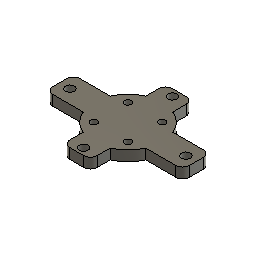
Base_Part1 (Autodesk Fusion 360 design; units mm, degrees)
part number: 2025-04-16-17-35-49-953
Autodesk Fusion 360 part; units mm, degrees
note: some values were not read from the file. Set by a fixed rule: which sketch regions a step uses.
sketch "Sketch1" plane through (0, 0, 0) normal (0, 1, 0) x (1, 0, 0)
  line L0 (20, 75) -> (-20, 75)
  line L1 (-100, 20) -> (-100, -20)
  line L2 (-20, -75) -> (20, -75)
  line L3 (100, -20) -> (100, 20)
  line L4 (20, 45.8258) -> (20, 75)
  line L5 (20, 75) -> (-20, 75)
  line L6 (-20, 75) -> (-20, 45.8258)
  line L7 (20, -45.8258) -> (20, -75)
  line L8 (20, -75) -> (-20, -75)
  line L9 (-20, -75) -> (-20, -45.8258)
  line L10 (45.8258, 20) -> (100, 20)
  line L11 (100, 20) -> (100, -20)
  line L12 (100, -20) -> (45.8258, -20)
  line L13 (-45.8258, 20) -> (-100, 20)
  line L14 (-100, 20) -> (-100, -20)
  arc A0 (45.8258, 20) -> (20, 45.8258) centre (0, 0) ccw
  arc A1 (-20, 45.8258) -> (-45.8258, 20) centre (0, 0) ccw
  line L15 (-100, -20) -> (-45.8258, -20)
  arc A2 (-45.8258, -20) -> (-20, -45.8258) centre (0, 0) ccw
  arc A3 (20, -45.8258) -> (45.8258, -20) centre (0, 0) ccw
  dimension "d70" = 100
  constraint horizontal L0
  constraint perpendicular L0 L1
  constraint parallel L0 L2
  constraint parallel L1 L3
  constraint coincident A0.centre A1.centre
  constraint vertical L4
  constraint horizontal L5
  constraint vertical L6
  constraint vertical L7
  constraint horizontal L8
  constraint vertical L9
  constraint horizontal L10
  constraint vertical L11
  constraint horizontal L12
  constraint horizontal L13
  constraint vertical L14
  constraint horizontal L15
  constraint coincident L10.start A1
  constraint concentric A0 A1
  constraint concentric A1 A2
  constraint concentric A2 A3
  measures "d70" diameter of A1
extrude "Extrude1" add sketch "Sketch1" along normal blind 15
sketch "Sketch3" plane through (0, 15, 0) normal (0, 1, 0) x (-1, 0, 0)
  line L0 (-20, 75) -> (-20, 45.8258)
  line L1 (-45.8258, 20) -> (-100, 20)
  line L2 (-100, 20) -> (-100, -20)
  line L3 (-100, -20) -> (-45.8258, -20)
  line L4 (-20, -45.8258) -> (-20, -75)
  line L5 (-20, -75) -> (20, -75)
  line L6 (20, -75) -> (20, -45.8258)
  line L7 (45.8258, -20) -> (100, -20)
  line L8 (100, -20) -> (100, 20)
  line L9 (100, 20) -> (45.8258, 20)
  line L10 (20, 45.8258) -> (20, 75)
  line L11 (20, 75) -> (-20, 75)
  circle A0 centre (0, 0) radius 50
  arc A1 (-20, 45.8258) -> (-45.8258, 20) centre (0, 0) ccw
  arc A2 (-45.8258, -20) -> (-20, -45.8258) centre (0, 0) ccw
  arc A3 (20, -45.8258) -> (45.8258, -20) centre (0, 0) ccw
  arc A4 (45.8258, 20) -> (20, 45.8258) centre (0, 0) ccw
  dimension "d71" = 100
  constraint coincident A0.centre A1.centre
  measures "d71" diameter of A0
sketch "Sketch4" plane through (0, 15, 0) normal (0, 1, 0) x (-1, 0, 0)
  line L0 (45.8258, -20) -> (100, -20)
  line L1 (100, -20) -> (100, 20)
  line L2 (100, 20) -> (45.8258, 20)
  circle A0 centre (0, -65) radius 6.5
  circle A1 centre (0, 65) radius 6.5
  circle A2 centre (-85, 0) radius 6.5
  circle A3 centre (85, 0) radius 6.5
  line L3 (-20, 75) -> (-20, 45.8258)
  arc A4 (-20, 45.8258) -> (-45.8258, 20) centre (0, 0) ccw
  line L4 (-45.8258, 20) -> (-100, 20)
  line L5 (-100, 20) -> (-100, -20)
  line L6 (-100, -20) -> (-45.8258, -20)
  arc A5 (-45.8258, -20) -> (-20, -45.8258) centre (0, 0) ccw
  line L7 (-20, -45.8258) -> (-20, -75)
  line L8 (-20, -75) -> (20, -75)
  line L9 (20, -75) -> (20, -45.8258)
  arc A6 (20, -45.8258) -> (45.8258, -20) centre (0, 0) ccw
  arc A7 (45.8258, 20) -> (20, 45.8258) centre (0, 0) ccw
  line L10 (20, 45.8258) -> (20, 75)
  line L11 (20, 75) -> (-20, 75)
  dimension "d30" = 13
  dimension "d31" = 13
  dimension "d32" = 13
  dimension "d33" = 13
  measures "d30" diameter of A0
  measures "d31" diameter of A1
  measures "d32" diameter of A2
  measures "d33" diameter of A3
extrude "Extrude3" cut sketch "Sketch4" against normal blind 15 contours A0 | A1 | A2 | A3
fillet "Fillet11" radius 10 1 edges at (20, 7.5, 75)
fillet "Fillet12" radius 10 7 edges at (100, 7.5, 20) (100, 7.5, -20) (20, 7.5, -75) (-100, 7.5, 20) (-20, 7.5, 75) (-20, 7.5, -75) (-100, 7.5, -20)
sketch "Sketch11" plane through (0, 15, 0) normal (0, 1, 0) x (-1, 0, 0)
  circle A0 centre (0, -65) radius 6.5
  circle A1 centre (-85, 0) radius 6.5
  circle A2 centre (85, 0) radius 6.5
  circle A3 centre (0, 65) radius 6.5
  arc A4 (90, -20) -> (100, -10) centre (90, -10) ccw
  line L0 (100, -10) -> (100, 10)
  arc A5 (100, 10) -> (90, 20) centre (90, 10) ccw
  line L1 (90, 20) -> (45.8258, 20)
  arc A6 (45.8258, 20) -> (20, 45.8258) centre (0, 0) ccw
  line L2 (20, 45.8258) -> (20, 65)
  arc A7 (20, 65) -> (10, 75) centre (10, 65) ccw
  line L3 (10, 75) -> (-10, 75)
  arc A8 (-10, 75) -> (-20, 65) centre (-10, 65) ccw
  line L4 (-20, 65) -> (-20, 45.8258)
  arc A9 (-20, 45.8258) -> (-45.8258, 20) centre (0, 0) ccw
  line L5 (-45.8258, 20) -> (-90, 20)
  arc A10 (-90, 20) -> (-100, 10) centre (-90, 10) ccw
  line L6 (-100, 10) -> (-100, -10)
  arc A11 (-100, -10) -> (-90, -20) centre (-90, -10) ccw
  line L7 (-90, -20) -> (-45.8258, -20)
  arc A12 (-45.8258, -20) -> (-20, -45.8258) centre (0, 0) ccw
  line L8 (-20, -45.8258) -> (-20, -65)
  arc A13 (-20, -65) -> (-10, -75) centre (-10, -65) ccw
  line L9 (-10, -75) -> (10, -75)
  arc A14 (10, -75) -> (20, -65) centre (10, -65) ccw
  line L10 (20, -65) -> (20, -45.8258)
  arc A15 (20, -45.8258) -> (45.8258, -20) centre (0, 0) ccw
  line L11 (45.8258, -20) -> (90, -20)
  line L12 (0, 0) -> (50, -50)
  line L13 (0, 0) -> (63.8718, 0) construction
  circle A16 centre (25, -25) radius 5
  circle A17 centre (25, 25) radius 5
  circle A18 centre (-25, 25) radius 5
  circle A19 centre (-25, -25) radius 5
  dimension "d77" = 45
  dimension "d78" = 10
  dimension "d79" = 25
  dimension "d81" = 360
  constraint horizontal L13
  constraint coincident A6.centre A9.centre
  constraint midpoint L12 A16.centre
  measures "d77" angle of L12 L13
  measures "d78" diameter of A16
  measures "d79" horizontal distance of A6.centre A16.centre
extrude "Extrude10" cut sketch "Sketch11" against normal blind 30 contours L12 A16 | L12 A16 | A17 | A18 | A19
sketch "Sketch12" plane through (0, 0, 0) normal (0, -1, 0) x (1, 0, 0)
  circle A0 centre (-25, -25) radius 5
  circle A1 centre (25, -25) radius 5
  circle A2 centre (-25, 25) radius 5
  circle A3 centre (25, 25) radius 5
  arc A4 (-100, -10) -> (-90, -20) centre (-90, -10) ccw
  line L0 (-90, -20) -> (-45.8258, -20)
  arc A5 (-45.8258, -20) -> (-20, -45.8258) centre (0, 0) ccw
  line L1 (-20, -45.8258) -> (-20, -65)
  arc A6 (-20, -65) -> (-10, -75) centre (-10, -65) ccw
  line L2 (-10, -75) -> (10, -75)
  arc A7 (10, -75) -> (20, -65) centre (10, -65) ccw
  line L3 (20, -65) -> (20, -45.8258)
  arc A8 (20, -45.8258) -> (45.8258, -20) centre (0, 0) ccw
  line L4 (45.8258, -20) -> (90, -20)
  arc A9 (90, -20) -> (100, -10) centre (90, -10) ccw
  line L5 (100, -10) -> (100, 10)
  arc A10 (100, 10) -> (90, 20) centre (90, 10) ccw
  line L6 (90, 20) -> (45.8258, 20)
  arc A11 (45.8258, 20) -> (20, 45.8258) centre (0, 0) ccw
  line L7 (20, 45.8258) -> (20, 65)
  arc A12 (20, 65) -> (10, 75) centre (10, 65) ccw
  line L8 (10, 75) -> (-10, 75)
  arc A13 (-10, 75) -> (-20, 65) centre (-10, 65) ccw
  line L9 (-20, 65) -> (-20, 45.8258)
  arc A14 (-20, 45.8258) -> (-45.8258, 20) centre (0, 0) ccw
  line L10 (-45.8258, 20) -> (-90, 20)
  arc A15 (-90, 20) -> (-100, 10) centre (-90, 10) ccw
  line L11 (-100, 10) -> (-100, -10)
  circle A16 centre (0, -65) radius 6.5
  circle A17 centre (85, 0) radius 6.5
  circle A18 centre (-85, 0) radius 6.5
  circle A19 centre (0, 65) radius 6.5
  line L12 (-29.9075, 33.5) -> (-34.815, 25)
  line L13 (-34.815, 25) -> (-29.9075, 16.5)
  line L14 (-29.9075, 16.5) -> (-20.0925, 16.5)
  line L15 (-20.0925, 16.5) -> (-15.185, 25)
  line L16 (-15.185, 25) -> (-20.0925, 33.5)
  line L17 (-20.0925, 33.5) -> (-29.9075, 33.5)
  line L18 (-16.5, -29.9075) -> (-16.5, -20.0925)
  line L19 (-25, -34.815) -> (-16.5, -29.9075)
  line L20 (-16.5, -20.0925) -> (-25, -15.185)
  circle A20 centre (-25, -25) radius 5
  line L21 (-25, -15.185) -> (-33.5, -20.0925)
  line L22 (-33.5, -29.9075) -> (-25, -34.815)
  line L23 (-33.5, -20.0925) -> (-33.5, -29.9075)
  line L24 (29.9075, -16.5) -> (20.0925, -16.5)
  line L25 (34.815, -25) -> (29.9075, -16.5)
  line L26 (20.0925, -16.5) -> (15.185, -25)
  circle A21 centre (25, -25) radius 5
  line L27 (15.185, -25) -> (20.0925, -33.5)
  line L28 (29.9075, -33.5) -> (34.815, -25)
  line L29 (20.0925, -33.5) -> (29.9075, -33.5)
  line L30 (16.5, 29.9075) -> (16.5, 20.0925)
  line L31 (25, 34.815) -> (16.5, 29.9075)
  line L32 (16.5, 20.0925) -> (25, 15.185)
  circle A22 centre (25, 25) radius 5
  line L33 (25, 15.185) -> (33.5, 20.0925)
  line L34 (33.5, 29.9075) -> (25, 34.815)
  line L35 (33.5, 20.0925) -> (33.5, 29.9075)
  point P0 (-25, 25)
  point P1 (-25, -25)
  point P2 (25, -25)
  point P3 (25, 25)
  dimension "d84" = 8.5
  dimension "d86" = 360
  constraint coincident P0 A2.centre
  measures "d84" distance of P0 L17
extrude "Extrude11" cut sketch "Sketch12" against normal blind 8 contours L12 L13 L14 L15 L16 L17 | L18 L19 L20 L21 L22 L23 | L24 L25 L26 L27 L28 L29 | L30 L31 L32 L33 L34 L35
sketch "Sketch5" plane through (0, 0, 0) normal (0, -1, 0) x (1, 0, 0)
  circle A0 centre (0, -65) radius 6.5
  circle A1 centre (85, 0) radius 6.5
  circle A2 centre (-85, 0) radius 6.5
  circle A3 centre (0, 65) radius 6.5
  arc A4 (-100, -10) -> (-90, -20) centre (-90, -10) ccw
  line L0 (-90, -20) -> (-45.8258, -20)
  line L1 (-20, -45.8258) -> (-20, -65)
  arc A5 (-20, -65) -> (-10, -75) centre (-10, -65) ccw
  line L2 (-10, -75) -> (10, -75)
  arc A6 (10, -75) -> (20, -65) centre (10, -65) ccw
  line L3 (20, -65) -> (20, -45.8258)
  line L4 (45.8258, -20) -> (90, -20)
  arc A7 (90, -20) -> (100, -10) centre (90, -10) ccw
  line L5 (100, -10) -> (100, 10)
  arc A8 (100, 10) -> (90, 20) centre (90, 10) ccw
  line L6 (90, 20) -> (45.8258, 20)
  line L7 (20, 45.8258) -> (20, 65)
  arc A9 (20, 65) -> (10, 75) centre (10, 65) ccw
  line L8 (10, 75) -> (-10, 75)
  arc A10 (-10, 75) -> (-20, 65) centre (-10, 65) ccw
  line L9 (-20, 65) -> (-20, 45.8258)
  line L10 (-45.8258, 20) -> (-90, 20)
  arc A11 (-90, 20) -> (-100, 10) centre (-90, 10) ccw
  line L11 (-100, 10) -> (-100, -10)
  circle A12 centre (0, 0) radius 22.5
  line L12 (25, 34.815) -> (33.5, 29.9075)
  line L13 (33.5, 29.9075) -> (33.5, 20.0925)
  line L14 (33.5, 20.0925) -> (25, 15.185)
  line L15 (25, 15.185) -> (16.5, 20.0925)
  line L16 (16.5, 20.0925) -> (16.5, 29.9075)
  line L17 (16.5, 29.9075) -> (25, 34.815)
  line L18 (34.815, -25) -> (29.9075, -33.5)
  line L19 (29.9075, -33.5) -> (20.0925, -33.5)
  line L20 (20.0925, -33.5) -> (15.185, -25)
  line L21 (15.185, -25) -> (20.0925, -16.5)
  line L22 (20.0925, -16.5) -> (29.9075, -16.5)
  line L23 (29.9075, -16.5) -> (34.815, -25)
  line L24 (-34.815, 25) -> (-29.9075, 33.5)
  line L25 (-29.9075, 33.5) -> (-20.0925, 33.5)
  line L26 (-20.0925, 33.5) -> (-15.185, 25)
  line L27 (-15.185, 25) -> (-20.0925, 16.5)
  line L28 (-20.0925, 16.5) -> (-29.9075, 16.5)
  line L29 (-29.9075, 16.5) -> (-34.815, 25)
  line L30 (-25, -34.815) -> (-33.5, -29.9075)
  line L31 (-33.5, -29.9075) -> (-33.5, -20.0925)
  line L32 (-33.5, -20.0925) -> (-25, -15.185)
  line L33 (-25, -15.185) -> (-16.5, -20.0925)
  line L34 (-16.5, -20.0925) -> (-16.5, -29.9075)
  line L35 (-16.5, -29.9075) -> (-25, -34.815)
  arc A13 (-45.8258, -20) -> (-20, -45.8258) centre (0, 0) ccw
  arc A14 (20, -45.8258) -> (45.8258, -20) centre (0, 0) ccw
  arc A15 (45.8258, 20) -> (20, 45.8258) centre (0, 0) ccw
  arc A16 (-20, 45.8258) -> (-45.8258, 20) centre (0, 0) ccw
  dimension "d72" = 45
  constraint coincident A12.centre A13.centre
  measures "d72" diameter of A12
extrude "Extrude4" cut sketch "Sketch5" against normal blind 10 contours A12
fillet "Fillet13" radius 5 1 edges at (-20.9774, 0, 8.1363)
equation "d84 = ( 17 / 2 ) * 1 mm"
